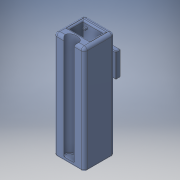
# Autodesk Inventor part: BaseStation
Saved by Autodesk Inventor 2016 (Build 200138000, 138)
## iProperties
Created: 2017-11-08
Part Number: BaseStation
Material: Generic
Document SubType Name: Modeling
Designer: kameo
Density: 1 g/cm^3
Appearance: Default
Author: kameo
## iProperties of the stored document BaseStation_3DPrint.ipt
Created: 2017-11-08
Part Number: BaseStation_3DPrint
Material: Generic
Document SubType Name: Modeling
Designer: kameo
Density: 1 g/cm^3
Appearance: Default
Author: kameo
Autodesk Inventor part; units mm, degrees
ref_plane "YZ Plane" through (0, 0, 0) normal (1, 0, 0) x (0, 1, 0)
ref_plane "XZ Plane" through (0, 0, 0) normal (0, 1, 0) x (-1, 0, 0)
ref_plane "XY Plane" through (0, 0, 0) normal (0, 0, 1) x (1, 0, 0)
sketch "Sketch1" plane through (0, 0, 0) normal (0, 1, 0) x (-1, 0, 0)
  line L0 (0, 0) -> (31.75, 0)
  line L1 (31.75, 0) -> (31.75, -31.75)
  line L2 (31.75, -31.75) -> (0, -31.75)
  line L3 (0, -31.75) -> (0, 0)
  dimension "d2" = 31.75
  dimension "d3" = 31.75
  constraints: 8 end point, 2 parallel, 1 horizontal, 1 perpendicular
  measures "d2" distance of L1.end L2.end
  measures "d3" distance of L0.end L1.end
extrude "Extrusion1" add sketch "Sketch1" along normal blind 111.76
sketch "Sketch2" plane through (0, 111.76, 0) normal (0, 1, 0) x (1, 0, 0)
  line L0 (-31.75, 0) -> (0, 0) projected
  ellipse E0 centre (-15.875, 3.175) end of major axis (-8.7186, 3.175) minor radius 4.8895
  line L1 (0, 0) -> (0, 31.75) projected
  dimension "d8" = 7.1565
  dimension "d9" = 4.8895
  dimension "d10" = 15.875
  dimension "d11" = 3.175
  constraints: 2 other
  measures "d10" distance from line of L1 point (-15.875, 3.175)
  measures "d11" distance from line of L0 point (-15.875, 3.175)
extrude "Extrusion2" cut sketch "Sketch2" against normal blind 107.95
sketch "Sketch3" plane through (0, 0, -31.75) normal (0, 0, -1) x (-1, 0, 0)
  line L0 (5.715, 0) -> (26.035, 0)
  line L1 (26.035, 0) -> (26.035, 50.8)
  line L2 (26.035, 50.8) -> (5.715, 50.8)
  line L3 (5.715, 50.8) -> (5.715, 0)
  line L4 (31.75, 0) -> (31.75, 111.76) projected
  line L5 (31.75, 0) -> (0, 0) projected
  dimension "d14" = 20.32
  dimension "d15" = 50.8
  dimension "d16" = 5.715
  constraints: 8 end point, 2 parallel, 1 collinear, 1 horizontal, 1 perpendicular
  measures "d14" distance of L2.end L1.end
  measures "d15" distance of L1.end L0.end
  measures "d16" distance between parallel lines of L4 L1
extrude "Extrusion3" cut sketch "Sketch3" against normal blind 2.54
sketch "Sketch4" plane through (0, 111.76, 0) normal (0, 1, 0) x (1, 0, 0)
  line L0 (-26.67, 10.795) -> (-5.08, 10.795)
  line L1 (-5.08, 10.795) -> (-5.08, 25.4)
  line L2 (-5.08, 25.4) -> (-26.67, 25.4)
  line L3 (-26.67, 25.4) -> (-26.67, 10.795)
  line L4 (-31.75, 0) -> (-31.75, 31.75) projected
  line L5 (0, 0) -> (0, 31.75) projected
  ellipse E0 centre (-15.875, 3.175) end of major axis (-23.0314, 3.175) minor radius 4.8895 (-10.4326, 0) -> (-21.3174, 0) ccw projected
  line L6 (0, 31.75) -> (-31.75, 31.75) projected
  dimension "d19" = 5.08
  dimension "d20" = 5.08
  dimension "d21" = 7.62
  dimension "d22" = 6.35
  constraints: 8 end point, 2 parallel, 1 horizontal, 1 perpendicular, 1 other
  measures "d19" distance between parallel lines of L4 L3
  measures "d20" distance between parallel lines of L5 L1
  measures "d21" distance from line of point (-15.875, 3.175) L0
  measures "d22" distance between parallel lines of L6 L2
extrude "Extrusion4" cut sketch "Sketch4" against normal blind 111.76
sketch "Sketch6" plane through (0, 0, -29.21) normal (0, 0, -1) x (-1, 0, 0)
  line L0 (5.715, 50.8) -> (26.035, 50.8)
  line L1 (26.035, 50.8) -> (26.035, 48.006)
  line L2 (26.035, 48.006) -> (5.715, 48.006)
  line L3 (5.715, 48.006) -> (5.715, 50.8)
  line L4 (5.715, 50.8) -> (26.035, 50.8) projected
  line L5 (5.715, 0) -> (5.715, 50.8) projected
  line L6 (26.035, 50.8) -> (26.035, 0) projected
  point P0 (0, 0)
  dimension "d25" = 2.794
  constraints: 8 end point, 3 collinear, 2 parallel, 1 horizontal, 1 perpendicular
  measures "d25" distance between parallel lines of L0 L2
extrude "Extrusion5" cut sketch "Sketch6" against normal blind 12.7
sketch "Sketch8" plane through (0, 0, 0) normal (0, -1, 0) x (1, 0, 0)
  line L0 (-26.67, -10.795) -> (-5.08, -10.795) projected
  line L1 (-5.08, -10.795) -> (-3.81, -10.795)
  line L2 (-3.81, -10.795) -> (-3.81, -12.3952)
  line L3 (-3.81, -12.3952) -> (-5.08, -12.3952)
  line L4 (-5.08, -12.3952) -> (-5.08, -10.795)
  line L5 (-26.67, -10.795) -> (-27.94, -10.795)
  line L6 (-27.94, -10.795) -> (-27.94, -12.3952)
  line L7 (-27.94, -12.3952) -> (-26.67, -12.3952)
  line L8 (-26.67, -12.3952) -> (-26.67, -10.795)
  point P0 (0, 0)
  dimension "d34" = 1.27
  dimension "d35" = 1.6002
  dimension "d36" = 1.27
  dimension "d37" = 1.6002
  constraints: 16 end point, 4 parallel, 2 horizontal, 2 perpendicular
  measures "d34" distance of L2.end L3.end
  measures "d35" distance of L1.end L2.end
  measures "d36" distance of L7.end L6.end
  measures "d37" distance of L6.end L5.end
extrude "Extrusion7" cut sketch "Sketch8" against normal blind 43.18
sketch "Sketch11" plane through (-26.67, 111.76, -25.4) normal (0, 0, 1) x (1, 0, 0)
  line L0 (16.764, -111.76) -> (21.59, -111.76)
  line L1 (21.59, -111.76) -> (21.59, -86.36)
  line L2 (21.59, -86.36) -> (16.764, -86.36)
  line L3 (16.764, -86.36) -> (16.764, -111.76)
  line L4 (21.59, -111.76) -> (0, -111.76) projected
  line L5 (0, 0) -> (0, -111.76) projected
  line L6 (21.59, 0) -> (21.59, -111.76) projected
  point P0 (26.67, -111.76)
  dimension "d50" = 25.4
  dimension "d51" = 16.764
  constraints: 8 end point, 2 collinear, 2 parallel, 1 horizontal, 1 perpendicular
  measures "d50" distance of L1.end L0.end
  measures "d51" distance between parallel lines of L5 L3
extrude "Extrusion10" add sketch "Sketch11" along normal blind 6.35
sketch "Sketch12" plane through (-9.906, 0, -25.4) normal (-1, 0, 0) x (0, 0, 1)
  line L0 (6.35, 25.4) -> (6.35, 0) projected
  line L1 (0, 0) -> (0, 25.4) projected
  line L2 (6.35, 4.953) -> (0, 4.953)
  line L3 (0, 4.953) -> (0, 3.175)
  line L4 (0, 3.175) -> (6.35, 3.175)
  line L5 (6.35, 3.175) -> (6.35, 4.953)
  line L6 (0, 0) -> (6.35, 0) projected
  point P0 (25.4, 0)
  dimension "d54" = 1.778
  dimension "d55" = 3.175
  constraints: 8 end point, 2 parallel, 2 point on line, 1 horizontal, 1 perpendicular
  measures "d54" distance between parallel lines of L4 L2
  measures "d55" distance between parallel lines of L6 L4
extrude "Extrusion11" cut sketch "Sketch12" against normal blind 2.54 contours L0 L4 L1 L2
sketch "Sketch13" plane through (-26.67, 111.76, -10.795) normal (1, 0, 0) x (0, 0, -1)
  line L0 (6.985, -111.76) -> (3.175, -111.76)
  line L1 (3.175, -111.76) -> (3.175, -86.36)
  line L2 (3.175, -86.36) -> (6.985, -86.36)
  line L3 (6.985, -86.36) -> (6.985, -111.76)
  line L4 (14.605, -111.76) -> (1.6002, -111.76) projected
  line L5 (14.605, 0) -> (14.605, -111.76) projected
  point P0 (-10.795, -111.76)
  dimension "d58" = 3.81
  dimension "d59" = 25.4
  dimension "d60" = 7.62
  constraints: 8 end point, 2 parallel, 1 collinear, 1 horizontal, 1 perpendicular
  measures "d58" distance of L1.end L2.end
  measures "d59" distance of L0.end L1.end
  measures "d60" distance between parallel lines of L3 L5
extrude "Extrusion12" cut sketch "Sketch13" against normal blind 1.27
draft "FaceDraft1" angle 2.85 pull direction (0, -1, 0) faces at (-27.94, 8.4667, -16.51) fixed edges at (-27.94, 0, -15.875)
sketch "Sketch14" plane through (-26.67, 111.76, -25.4) normal (0, 0, 1) x (1, 0, 0)
  circle A0 centre (18.295, -5.31) radius 1.5
  circle A1 centre (3.295, -5.31) radius 1.5
  line L0 (18.295, -5.31) -> (3.295, -5.31) construction
  line L1 (0, 0) -> (21.59, 0) construction
  line L2 (0, 0) -> (0, -111.76) construction
  point P0 (26.67, -111.76)
  dimension "d64" = 3
  dimension "d65" = 3
  dimension "d66" = 15
  dimension "d67" = 3.295
  dimension "d68" = 5.31
  constraints: 2 centre point, 2 end point, 1 parallel
  measures "d64" diameter of A0
  measures "d65" diameter of A1
  measures "d66" distance of L0.end L0.start
  measures "d67" distance from line of L2 L0.end
  measures "d68" distance from line of L1 L0.end
extrude "Extrusion13" add sketch "Sketch14" along normal blind 2.54
sketch "Sketch15" plane through (0, 111.76, -31.75) normal (0, 0, -1) x (-1, 0, 0)
  line L0 (12.7, -50.8) -> (19.05, -50.8)
  line L1 (19.05, -50.8) -> (19.05, -25.4)
  line L2 (19.05, -25.4) -> (12.7, -25.4)
  line L3 (12.7, -25.4) -> (12.7, -50.8)
  line L4 (31.75, -111.76) -> (31.75, 0) projected
  line L5 (26.67, 0) -> (5.08, 0) projected
  point P0 (0, -111.76)
  dimension "d71" = 6.35
  dimension "d72" = 25.4
  dimension "d73" = 12.7
  dimension "d74" = 25.4
  constraints: 8 end point, 2 parallel, 1 horizontal, 1 perpendicular
  measures "d71" distance of L2.end L1.end
  measures "d72" distance of L1.end L0.end
  measures "d73" distance between parallel lines of L4 L1
  measures "d74" distance between parallel lines of L5 L2
extrude "Extrusion14" add sketch "Sketch15" along normal blind 12.7
sketch "Sketch16" plane through (-12.7, 60.96, -31.75) normal (1, 0, 0) x (0, 0, -1)
  line L0 (0, 25.4) -> (12.7, 25.4) projected
  line L1 (12.7, 0) -> (7.62, 0)
  line L2 (7.62, 0) -> (7.62, 25.4)
  line L3 (7.62, 25.4) -> (12.7, 25.4)
  line L4 (12.7, 25.4) -> (12.7, 0)
  point P0 (-31.75, -60.96)
  dimension "d77" = 5.08
  constraints: 8 end point, 2 parallel, 1 horizontal, 1 perpendicular, 1 point on line
  measures "d77" distance between parallel lines of L4 L2
extrude "Extrusion15" add sketch "Sketch16" along normal blind 6.35
sketch "Sketch17" plane through (-19.05, 60.96, -31.75) normal (-1, 0, 0) x (0, 0, 1)
  line L0 (-12.7, 0) -> (-12.7, 25.4) projected
  line L1 (0, 0) -> (-12.7, 0) projected
  line L2 (-12.7, 25.4) -> (-7.62, 25.4)
  line L3 (-7.62, 25.4) -> (-7.62, 0)
  line L4 (-7.62, 0) -> (-12.7, 0)
  line L5 (-12.7, 0) -> (-12.7, 25.4)
  point P0 (31.75, -60.96)
  dimension "d80" = 5.08
  constraints: 8 end point, 2 parallel, 1 horizontal, 1 perpendicular, 1 point on line
  measures "d80" distance of L3.end L4.end
extrude "Extrusion16" add sketch "Sketch17" along normal blind 6.35
fillet "Fillet1" radius 3.175 1 edges at (0, 55.88, -31.75)
fillet "Fillet2" radius 3.175 3 edges at (-31.75, 55.88, -31.75) (-31.75, 55.88, 0) (0, 55.88, 0)
fillet "Fillet3" radius 3.175 9 edges at (-0.9299, 111.76, -30.8201) (-15.875, 111.76, -31.75) (-30.8201, 111.76, -30.8201) (-31.75, 111.76, -15.875) (-30.8201, 111.76, -0.9299) (-24.9462, 111.76, 0) (-0.9299, 111.76, -0.9299) (-6.8038, 111.76, 0) (0, 111.76, -15.875)
fillet "Fillet4" radius 1.5875 4 edges at (-26.67, 111.76, -18.0975) (-15.875, 111.76, -10.795) (-5.08, 111.76, -18.0975) (-15.875, 111.76, -25.4)
fillet "Fillet5" radius 1.5875 9 edges at (-0.9299, 0, -0.9299) (-15.875, 0, 0) (-30.8201, 0, -0.9299) (-31.75, 0, -15.875) (-30.8201, 0, -30.8201) (-27.305, 0, -31.75) (-0.9299, 0, -30.8201) (-4.445, 0, -31.75) (0, 0, -15.875)
fillet "Fillet6" radius 0.762 4 edges at (-6.35, 73.66, -44.45) (-25.4, 73.66, -44.45) (-6.35, 73.66, -39.37) (-25.4, 73.66, -39.37)
fillet "Fillet7" radius 0.762 9 edges at (-25.1768, 60.96, -39.5932) (-21.844, 60.96, -39.37) (-25.1768, 60.96, -44.2268) (-15.875, 60.96, -44.45) (-6.5732, 60.96, -44.2268) (-6.35, 60.96, -41.91) (-6.5732, 60.96, -39.5932) (-9.906, 60.96, -39.37) (-25.4, 60.96, -41.91)
fillet "Fillet8" radius 0.762 9 edges at (-25.1768, 86.36, -44.2268) (-15.875, 86.36, -44.45) (-6.5732, 86.36, -44.2268) (-6.35, 86.36, -41.91) (-6.5732, 86.36, -39.5932) (-9.906, 86.36, -39.37) (-25.1768, 86.36, -39.5932) (-21.844, 86.36, -39.37) (-25.4, 86.36, -41.91)
fillet "Fillet9" radius 0.762 2 edges at (-18.3515, 3.81, -7.7624) (-9.1607, 3.81, -1.483)
fillet "Fillet10" radius 0.762 1 edges at (-9.875, 106.45, -22.86)
fillet "Fillet11" radius 0.762 1 edges at (-24.875, 106.45, -22.86)
fillet "Fillet12" radius 0.762 2 edges at (-19.05, 86.36, -39.751) (-19.05, 86.36, -35.56)
fillet "Fillet13" radius 0.762 2 edges at (-12.7, 86.36, -35.56) (-12.7, 86.36, -39.751)
fillet "Fillet14" radius 0.762 4 edges at (-19.05, 60.96, -35.56) (-19.05, 60.96, -39.751) (-12.7, 60.96, -35.56) (-12.7, 60.96, -39.751)
body "Solid1"
